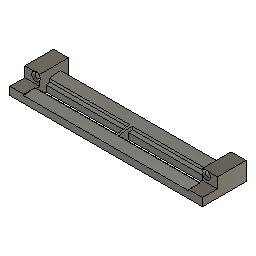
led_pcb_mount (Autodesk Fusion 360 design; units mm, degrees)
Autodesk Fusion 360 part; units mm, degrees
sketch "Sketch1" plane through (0, 0, 0) normal (0, 0, 1) x (1, 0, 0)
  line L0 (0, 0) -> (84, 0)
  line L1 (84, 0) -> (84, 38)
  line L2 (84, 38) -> (0, 38)
  line L3 (0, 38) -> (0, 0)
  line L4 (71, 38) -> (84, 38)
  line L5 (84, 38) -> (84, 31)
  line L6 (84, 31) -> (71, 31)
  line L7 (71, 31) -> (71, 38)
  line L8 (71, 31) -> (0, 31)
  line L9 (0, 31) -> (0, 38)
  line L10 (0, 38) -> (71, 38)
  line L11 (71, 38) -> (71, 31)
  line L12 (1, 31) -> (72, 31)
  line L13 (72, 31) -> (72, 0)
  line L14 (72, 0) -> (1, 0)
  line L15 (1, 0) -> (1, 31)
  line L16 (1, 18.5) -> (72, 18.5)
  line L17 (72, 18.5) -> (72, 12.5)
  line L18 (72, 12.5) -> (1, 12.5)
  line L19 (1, 12.5) -> (1, 18.5)
  dimension "d1" = 84
  dimension "d2" = 13
  dimension "d3" = 7
  dimension "d4" = 38
  dimension "d5" = 1
  dimension "d6" = 71
  dimension "d7" = 6
  dimension "d8" = 12.5
  constraint horizontal L0
  constraint vertical L1
  constraint horizontal L2
  constraint vertical L3
  constraint coincident L0.start L3.end
  constraint horizontal L4
  constraint vertical L5
  constraint horizontal L6
  constraint vertical L7
  constraint coincident L1 L5.end
  constraint coincident L2 L4.start
  constraint horizontal L8
  constraint vertical L9
  constraint horizontal L10
  constraint vertical L11
  constraint horizontal L12
  constraint vertical L13
  constraint horizontal L14
  constraint vertical L15
  constraint coincident L0 L13.end
  constraint coincident L8 L12.start
  constraint horizontal L16
  constraint vertical L17
  constraint horizontal L18
  constraint vertical L19
  constraint coincident L13 L17.end
  constraint coincident L15 L16.start
  measures "d1" distance of L1 L3
  measures "d2" distance of L5 L7
  measures "d3" distance of L4 L6
  measures "d4" distance of L0 L2
  measures "d5" distance of L3 L15
  measures "d6" distance of L13 L15
  measures "d7" distance of L16 L18
  measures "d8" distance of L0 L18
extrude "Extrude1" add sketch "Sketch1" along normal blind 16 contours L0 L3 L8 L15 L19 | L0 L1 L6 L13 L17 | L1 L2 L4 L5 L6 L7 L11 L12 makes body 1 at (84, 12.6667, 5.3333) makes body 2 at (0, 20.6667, 5.3333)
extrude "Extrude2" add sketch "Sketch1" along normal blind 10 contours L0 L13 L14 L15 L18 | L6 L8 L12 L13 L15 L16 bodies 1 2
sketch "Sketch3" plane through (72, 0, 0) normal (-1, 0, 0) x (0, -1, 0)
  line L0 (0, 16) -> (-31, 16)
  line L1 (-18.5, 10) -> (-18.5, 0)
  line L2 (-18.5, 0) -> (-12.5, 0)
  line L3 (-12.5, 0) -> (-12.5, 10)
  line L4 (-31, 10) -> (-31, 0)
  line L5 (0, 10) -> (0, 0)
  line L6 (-31, 10) -> (0, 6)
  line L7 (-12.5, 10) -> (0, 10)
  line L8 (0, 10) -> (0, 16)
  line L9 (-31, 16) -> (-31, 10)
  line L10 (-31, 10) -> (-18.5, 10)
  point P0 (-31, 0)
  dimension "d13" = 10
  dimension "d14" = 4
  constraint coincident L5.end origin
  constraint coincident L5 L6.end
  constraint coincident P0 L4.end
  constraint equal L4 L5
  measures "d13" distance of L4.start P0
  measures "d14" distance of L5.start L6.end
extrude "Extrude3" cut sketch "Sketch3" along normal blind 72 contours L0 L1 L3 L6 L7 L8 L9 L10 | L3 L5 L6 L7 | L1 L6 L10 bodies 1
sketch "Sketch4" plane through (0, 0, 16) normal (0, 0, 1) x (-1, 0, 0)
  line L0 (-71, -38) -> (-71, -31)
  line L1 (-72, -13) -> (-72, 0)
  line L2 (-72, 0) -> (-84, 0)
  line L3 (-84, 0) -> (-84, -38)
  line L4 (-84, -38) -> (-71, -38)
  line L5 (-72, -13) -> (-84, -13)
  line L6 (-84, -13) -> (-84, 0)
  line L7 (-84, 0) -> (-72, 0)
  line L8 (-72, 0) -> (-72, -31)
  line L9 (-71, -31) -> (-72, -31)
  line L10 (-84, -38) -> (0, -38)
  dimension "d32" = 25
  constraint horizontal L5
  constraint vertical L6
  constraint horizontal L7
  constraint vertical L8
  constraint coincident L2.end L3.start
  constraint coincident L8.end L9.end
  constraint coincident L8 L1.start
  measures "d32" distance of L5 L10
extrude "Extrude4" cut sketch "Sketch4" against normal blind 9 contours L1 L2 L3 L5 L6 L7 L8 bodies 1
sketch "Sketch5" plane through (0, 31, 0) normal (0, -1, 0) x (1, 0, 0)
  line L0 (71, 10) -> (72, 10)
  line L1 (72, 7) -> (84, 7)
  line L2 (84, 7) -> (84, 16)
  line L3 (72, 16) -> (71, 16)
  line L4 (71, 16) -> (71, 10)
  line L5 (71, 12.75) -> (84, 12.75)
  circle A0 centre (74.25, 12.75) radius 2.25
  line L6 (72, 10) -> (72, 16)
  line L7 (84, 16) -> (72, 16)
  line L8 (72, 16) -> (72, 7)
  dimension "d19" = 3.25
  dimension "d20" = 4.5
  dimension "d21" = 3.25
  constraint coincident L4 L5.start
  constraint coincident L2 L5.end
  constraint perpendicular L2 L5
  constraint coincident L5 A0.centre
  measures "d19" distance of L3 L5
  measures "d20" diameter of A0
  measures "d21" distance of L5.start A0.centre
extrude "Extrude5" cut sketch "Sketch5" against normal blind 7 contours L5 A0 | L5 A0 bodies 1
sketch "Sketch6" plane through (0, -0.7615, 5.9017) normal (0, -0.127971, 0.991778) x (1, 0, 0)
  line L0 (72, 13.3715) -> (1, 13.3715)
  line L1 (1, 13.3715) -> (1, 19.4212)
  line L2 (1, 19.4212) -> (72, 19.4212)
  line L3 (72, 32.0248) -> (71, 32.0248)
  line L4 (71, 32.0248) -> (0, 32.0248)
  line L5 (0, 32.0248) -> (0, 0.7678)
  line L6 (0, 0.7678) -> (72, 0.7678)
  line L7 (72, 8.5821) -> (72, 13.3715)
  line L8 (1, 19.4212) -> (72, 19.4212)
  line L9 (72, 19.4212) -> (72, 22.4212)
  line L10 (72, 22.4212) -> (1, 22.4212)
  line L11 (1, 22.4212) -> (1, 19.4212)
  line L12 (1, 13.3715) -> (72, 13.3715)
  line L13 (72, 13.3715) -> (72, 10.3715)
  line L14 (72, 10.3715) -> (1, 10.3715)
  line L15 (1, 10.3715) -> (1, 13.3715)
  line L16 (1, 19.4212) -> (72, 19.4212)
  line L17 (72, 19.4212) -> (72, 13.3715)
  line L18 (72, 13.3715) -> (1, 13.3715)
  line L19 (1, 13.3715) -> (1, 19.4212)
  line L20 (72, 19.4212) -> (72, 32.0248)
  line L21 (72, 0.7678) -> (72, 8.5821)
  dimension "d26" = 3
  dimension "d27" = 3
  constraint horizontal L8
  constraint vertical L9
  constraint horizontal L10
  constraint vertical L11
  constraint coincident L1.end L2.start
  constraint horizontal L12
  constraint vertical L13
  constraint horizontal L14
  constraint vertical L15
  constraint coincident L7 L13.end
  constraint coincident L0.end L1.start
  constraint horizontal L16
  constraint vertical L17
  constraint horizontal L18
  constraint vertical L19
  measures "d26" distance of L8 L10
  measures "d27" distance of L12 L14
extrude "Extrude6" cut sketch "Sketch6" against normal blind 3 contours L0 L7 L12 L13 L14 L15 L18 | L0 L1 L2 L8 L12 L16 L17 L18 L19 | L2 L8 L9 L10 L11 L16 L20 bodies 1
extrude "Extrude7" cut 1 faces at (73.7002, 31, 11.7977) along direction (0, -1, 0) blind 18 on bodies 1 bodies 1
extrude "Extrude10" add 1 faces at (71.3333, 31, 12.9167) along direction (0, -1, 0) blind 18 on bodies 1 bodies 1
extrude "Extrude11" add 1 faces at (71.3333, 25, 10) along direction (0, 0, -1) blind 10 on bodies 1 bodies 1
extrude "Extrude12" add 1 faces at (72, 11.6847, 6.196) along direction (-1, 0, 0) blind 1 on bodies 1 bodies 1
chamfer "Chamfer2" distance 1.5 angle 45 1 edges at (72.1523, 13, 13.5636) on bodies 1
mirror "Mirror2" about plane through (0, 31, 0) normal (-1, 0, 0) of bodies 1 merged
sketch "Sketch8" plane through (71, 0, 0) normal (-1, 0, 0) x (0, -1, 0)
  spline S0 degree 2 poles (-13, 14.6208) (-13.9333, 12.75) (-13, 10.8792) knots 0.425877 0.425877 0.425877 1.081253 1.081253 1.081253 weights 1.492255 1.721833 1.492255
  line L0 (-13, 14.6208) -> (-13, 16)
  line L1 (-13, 16) -> (-38, 16)
  line L2 (-38, 16) -> (-38, 0)
  line L3 (-38, 0) -> (-31, 0)
  line L4 (-31, 0) -> (-31, 10)
  line L5 (-31, 10) -> (-21.4753, 8.771)
  line L6 (-21.4753, 8.771) -> (-21.8592, 5.7957)
  line L7 (-21.8592, 5.7957) -> (-18.5, 5.3622)
  line L8 (-18.5, 5.3622) -> (-18.5, 0)
  line L9 (-18.5, 0) -> (-12.5, 0)
  line L10 (-12.5, 0) -> (-12.5, 4.588)
  line L11 (-12.5, 4.588) -> (-9.9086, 4.2537)
  line L12 (-9.9086, 4.2537) -> (-9.5542, 7)
  line L13 (-9.5542, 7) -> (-13, 7)
  line L14 (-13, 7) -> (-13, 10.8792)
